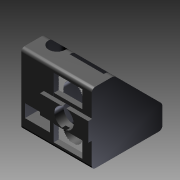
# Autodesk Inventor part: May Tec 1.64.153030.2_Mounting blocks GD-Zn_schwarz 0
Saved by Autodesk Inventor 2016 (Build 200138000, 138)
## iProperties
Category: PARTsolutions
Company: MAYTEC
Created: 2012-11-14
Part Number: May Tec 1.64.153030.2_Mounting blocks GD-Zn_schwarz 0
Catalog Web Link: www.cadenas.de
Description: 1.64.153030-Mounting block
Vendor: MAYTEC
Document SubType Name: Modeling
Designer: PARTuser1
Manufacturer: MAYTEC
Density: 1 g/cm^3
Material: Generic
Appearance: RGB(0.00000000000000,0.00000000000000,0.00000000000000)
Mass: 10.5528 g
Surface Area: 72.8477 cm^2
Volume: 10.5528 cm^3
PSOL_IDENT_0: {\\10.0.0.242\data_v9\23d-libs\maytec\maytec_3d\anbauzubehoer\befestigungsbloecke\befestigungsblock_
PSOL_IDENT_1: gd-zn.prj},254 {VTYP=3D},{NB=May Tec 1.64.153030.2_Mounting blocks GD-Zn_schwarz 0},{LINA=May Tec 1.
PSOL_IDENT_2: 64.153030.2_Mounting blocks GD-Zn_schwarz 0},{NN=1.64.153030},{DATE=14.09.2010 08:30:06},{GEOMDATE=0
PSOL_IDENT_3: 6.07.2009 00:00:00},{VERSION=},{LINEID=20},{LINESUBID=-1},{WBVAR=P}  {NB=May Tec 1.64.153030.2_Mount
PSOL_IDENT_4: ing blocks GD-Zn_schwarz 0},{LINA=May Tec 1.64.153030.2_Mounting blocks GD-Zn_schwarz 0},{KT=DUMMY},
PSOL_IDENT_5: {PARTNR=1.64.153030.2},{DESCRIPTION=Befestigungsblock GD-Zn},{B=30.0},{H=30.0},{L=30.0},{COLOR=schwa
PSOL_IDENT_6: rz},{COL=0.00,0.00,0.00,0.00},{XTRANS=Mounting blocks GD-Zn},{P=0}
CNS_NT: Mounting block
CNS_NB: May Tec 1.64.153030.2_Mounting blocks GD-Zn_schwarz 0
CNS_NBSYN: May Tec $PARTNR._$XTRANS._$COLOR. $P.
CNS_LINA: May Tec 1.64.153030.2_Mounting blocks GD-Zn_schwarz 0
CNS_PARTNR: 1.64.153030.2
CNS_DESCRIPTION: Mounting blocks GD-Zn
CNS_B: 30.0
CNS_H: 30.0
CNS_L: 30.0
CNS_COLOR: Black
CNS_COL: 0.00,0.00,0.00,0.00
CNS_XTRANS: Mounting blocks GD-Zn
CNS_P: 0
SUPPLIER: MAYTEC
ARTICLENO: May Tec 1.64.153030.2_Mounting blocks GD-Zn_schwarz 0
BOMINFO: May Tec 1.64.153030.2_Mounting blocks GD-Zn_schwarz 0
CREATOR: CADENAS GmbH
Title: May Tec 1.64.153030.2_Mounting blocks GD-Zn_schwarz 0
Author: Cadenas PARTsolutions
Comments: Mounting block
Autodesk Inventor part; units mm, degrees
sketch "Skizze_1" plane through (0, 0, 0) normal (1, 0, 0) x (0, 1, 0)
  arc A0 (1.5, 30) -> (0, 28.5) centre (1.5, 28.5) ccw
  line L0 (0, 28.5) -> (0, 1.5)
  arc A1 (0, 1.5) -> (1.5, 0) centre (1.5, 1.5) ccw
  line L1 (1.5, 0) -> (28.5, 0)
  arc A2 (28.5, 0) -> (30, 1.5) centre (28.5, 1.5) ccw
  line L2 (30, 1.5) -> (30, 8.4645)
  arc A3 (30, 8.4645) -> (29.2678, 10.2322) centre (27.5, 8.4645) ccw
  line L3 (29.2678, 10.2322) -> (10.2322, 29.2678)
  arc A4 (10.2322, 29.2678) -> (8.4645, 30) centre (8.4645, 27.5) ccw
  line L4 (8.4645, 30) -> (1.5, 30)
  constraints: 10 end point, 10 point on circle, 5 centre point
extrude "Extrusion1" add sketch "Skizze_1" along normal mid plane 30
sketch "Sketch2" plane through (15, 1.5, 0) normal (0, 0, -1) x (-1, 0, 0)
  point P0 (23.5, 21)
hole "Drilling 1" at (-8.5, 22.5, 0) direction (0, 0, 1) diameter 6.647 depth 12 countersink diameter 8 countersink angle 90 thread size "M8x1.25" class "6H" standard "ISO Metric profile"
sketch "Sketch3" plane through (-8.5, 22.5, 12) normal (0, 0, -1) x (-1, 0, 0)
  point P0 (0, 0)
hole "Drilling 2" at (-8.5, 22.5, 12) direction (0, 0, 1) diameter 10 depth 13
sketch "Skizze_5" plane through (0, 0, 30) normal (0, 0, 1) x (1, 0, 0)
  arc A0 (-12, 8.7) -> (-5, 8.7) centre (-8.5, 8.7) ccw
  line L0 (-5, 8.7) -> (-5, 12.9)
  arc A1 (-5, 12.9) -> (-12, 12.9) centre (-8.5, 12.9) ccw
  line L1 (-12, 12.9) -> (-12, 8.7)
  constraints: 4 end point, 4 point on circle, 2 centre point
extrude "Extrusion2" cut sketch "Skizze_5" against normal blind 30
sketch "Skizze_4" plane through (0, 0, 30) normal (0, 0, 1) x (1, 0, 0)
  line L0 (-2.4, 8) -> (12.1, 8)
  line L1 (12.1, 8) -> (12.1, 38)
  line L2 (12.1, 38) -> (-2.4, 38)
  line L3 (-2.4, 38) -> (-2.4, 8)
  constraints: 8 end point
extrude "Extrusion3" cut sketch "Skizze_4" against normal blind 24.1
sketch "Skizze_6" plane through (0, 0, 30) normal (0, 0, 1) x (1, 0, 0)
  arc A0 (0.75, 15.6) -> (8.95, 15.6) centre (4.85, 15.6) ccw
  line L0 (8.95, 15.6) -> (8.95, 20.6)
  arc A1 (8.95, 20.6) -> (0.75, 20.6) centre (4.85, 20.6) ccw
  line L1 (0.75, 20.6) -> (0.75, 15.6)
  constraints: 4 end point, 4 point on circle, 2 centre point
extrude "Extrusion4" cut sketch "Skizze_6" against normal blind 30
sketch "Skizze_8" plane through (0, 8, 0) normal (0, 1, 0) x (1, 0, 0)
  line L0 (4.9, -8) -> (4.9, -1)
  arc A0 (12, -8) -> (4.9, -1) centre (4.8281, -8.1737) ccw
  line L1 (12, -8) -> (4.9, -8)
  line L2 (4.9, -8) -> (4.9, -1)
  constraints: 6 end point, 2 point on circle, 1 centre point
revolve "Revolution1" cut sketch "Skizze_8" angle 180 about axis through (4.9, 8, 8) along (0, 0, 1)
sketch "Skizze_9" plane through (0, 0, 0) normal (0, 1, 0) x (-1, 0, 0)
  arc A0 (-0.8, 22.15) -> (-9, 22.15) centre (-4.9, 22.15) ccw
  line L0 (-9, 22.15) -> (-9, 7.85)
  arc A1 (-9, 7.85) -> (-0.8, 7.85) centre (-4.9, 7.85) ccw
  line L1 (-0.8, 7.85) -> (-0.8, 22.15)
  constraints: 4 end point, 4 point on circle, 2 centre point
extrude "Extrusion5" cut sketch "Skizze_9" along normal blind 30
sketch "Skizze_10" plane through (0, 0, 0) normal (0, 1, 0) x (-1, 0, 0)
  line L0 (1.2, 27.8) -> (-11, 27.8)
  line L1 (-11, 27.8) -> (-11, 2.2)
  line L2 (-11, 2.2) -> (1.2, 2.2)
  line L3 (1.2, 2.2) -> (1.2, 27.8)
  constraints: 8 end point
extrude "Extrusion6" cut sketch "Skizze_10" along normal blind 2
sketch "Skizze_11" plane through (0, 0, 0) normal (0, 1, 0) x (-1, 0, 0)
  line L0 (13.4, 5) -> (13.4, 10.5)
  line L1 (13.4, 10.5) -> (2.75, 10.5)
  line L2 (2.75, 10.5) -> (2.75, 5)
  line L3 (2.75, 5) -> (13.4, 5)
  constraints: 8 end point
extrude "Extrusion7" cut sketch "Skizze_11" along normal blind 17.65
sketch "Skizze_7" plane through (4.9, 0, 0) normal (1, 0, 0) x (0, 0, -1)
  line L0 (-27.8, 1.7273) -> (-2.2, 1.7273)
  line L1 (-2.2, 1.7273) -> (-2.2, 2.3)
  line L2 (-2.2, 2.3) -> (-2.5, 2)
  line L3 (-2.5, 2) -> (-2.75, 2.3)
  line L4 (-2.75, 2.3) -> (-3, 2)
  line L5 (-3, 2) -> (-3.25, 2.3)
  line L6 (-3.25, 2.3) -> (-3.5, 2)
  line L7 (-3.5, 2) -> (-3.75, 2.3)
  line L8 (-3.75, 2.3) -> (-4, 2)
  line L9 (-4, 2) -> (-4.25, 2.3)
  line L10 (-4.25, 2.3) -> (-4.5, 2)
  line L11 (-4.5, 2) -> (-4.75, 2.3)
  line L12 (-4.75, 2.3) -> (-5, 2)
  line L13 (-5, 2) -> (-5.25, 2.3)
  line L14 (-5.25, 2.3) -> (-5.5, 2)
  line L15 (-5.5, 2) -> (-5.75, 2.3)
  line L16 (-5.75, 2.3) -> (-6, 2)
  line L17 (-6, 2) -> (-6.25, 2.3)
  line L18 (-6.25, 2.3) -> (-6.5, 2)
  line L19 (-6.5, 2) -> (-6.75, 2.3)
  line L20 (-6.75, 2.3) -> (-7, 2)
  line L21 (-7, 2) -> (-7.25, 2.3)
  line L22 (-7.25, 2.3) -> (-7.5, 2)
  line L23 (-7.5, 2) -> (-7.75, 2.3)
  line L24 (-7.75, 2.3) -> (-8, 2)
  line L25 (-8, 2) -> (-8.25, 2.3)
  line L26 (-8.25, 2.3) -> (-8.5, 2)
  line L27 (-8.5, 2) -> (-8.75, 2.3)
  line L28 (-8.75, 2.3) -> (-9, 2)
  line L29 (-9, 2) -> (-9.25, 2.3)
  line L30 (-9.25, 2.3) -> (-9.5, 2)
  line L31 (-9.5, 2) -> (-9.75, 2.3)
  line L32 (-9.75, 2.3) -> (-10, 2)
  line L33 (-10, 2) -> (-10.25, 2.3)
  line L34 (-10.25, 2.3) -> (-10.5, 2)
  line L35 (-10.5, 2) -> (-10.75, 2.3)
  line L36 (-10.75, 2.3) -> (-11, 2)
  line L37 (-11, 2) -> (-11.25, 2.3)
  line L38 (-11.25, 2.3) -> (-11.5, 2)
  line L39 (-11.5, 2) -> (-11.75, 2.3)
  line L40 (-11.75, 2.3) -> (-12, 2)
  line L41 (-12, 2) -> (-12.25, 2.3)
  line L42 (-12.25, 2.3) -> (-12.5, 2)
  line L43 (-12.5, 2) -> (-12.75, 2.3)
  line L44 (-12.75, 2.3) -> (-13, 2)
  line L45 (-13, 2) -> (-13.25, 2.3)
  line L46 (-13.25, 2.3) -> (-13.5, 2)
  line L47 (-13.5, 2) -> (-13.75, 2.3)
  line L48 (-13.75, 2.3) -> (-14, 2)
  line L49 (-14, 2) -> (-14.25, 2.3)
  line L50 (-14.25, 2.3) -> (-14.5, 2)
  line L51 (-14.5, 2) -> (-14.75, 2.3)
  line L52 (-14.75, 2.3) -> (-15, 2)
  line L53 (-15, 2) -> (-15.25, 2.3)
  line L54 (-15.25, 2.3) -> (-15.5, 2)
  line L55 (-15.5, 2) -> (-15.75, 2.3)
  line L56 (-15.75, 2.3) -> (-16, 2)
  line L57 (-16, 2) -> (-16.25, 2.3)
  line L58 (-16.25, 2.3) -> (-16.5, 2)
  line L59 (-16.5, 2) -> (-16.75, 2.3)
  line L60 (-16.75, 2.3) -> (-17, 2)
  line L61 (-17, 2) -> (-17.25, 2.3)
  line L62 (-17.25, 2.3) -> (-17.5, 2)
  line L63 (-17.5, 2) -> (-17.75, 2.3)
  line L64 (-17.75, 2.3) -> (-18, 2)
  line L65 (-18, 2) -> (-18.25, 2.3)
  line L66 (-18.25, 2.3) -> (-18.5, 2)
  line L67 (-18.5, 2) -> (-18.75, 2.3)
  line L68 (-18.75, 2.3) -> (-19, 2)
  line L69 (-19, 2) -> (-19.25, 2.3)
  line L70 (-19.25, 2.3) -> (-19.5, 2)
  line L71 (-19.5, 2) -> (-19.75, 2.3)
  line L72 (-19.75, 2.3) -> (-20, 2)
  line L73 (-20, 2) -> (-20.25, 2.3)
  line L74 (-20.25, 2.3) -> (-20.5, 2)
  line L75 (-20.5, 2) -> (-20.75, 2.3)
  line L76 (-20.75, 2.3) -> (-21, 2)
  line L77 (-21, 2) -> (-21.25, 2.3)
  line L78 (-21.25, 2.3) -> (-21.5, 2)
  line L79 (-21.5, 2) -> (-21.75, 2.3)
  line L80 (-21.75, 2.3) -> (-22, 2)
  line L81 (-22, 2) -> (-22.25, 2.3)
  line L82 (-22.25, 2.3) -> (-22.5, 2)
  line L83 (-22.5, 2) -> (-22.75, 2.3)
  line L84 (-22.75, 2.3) -> (-23, 2)
  line L85 (-23, 2) -> (-23.25, 2.3)
  line L86 (-23.25, 2.3) -> (-23.5, 2)
  line L87 (-23.5, 2) -> (-23.75, 2.3)
  line L88 (-23.75, 2.3) -> (-24, 2)
  line L89 (-24, 2) -> (-24.25, 2.3)
  line L90 (-24.25, 2.3) -> (-24.5, 2)
  line L91 (-24.5, 2) -> (-24.75, 2.3)
  line L92 (-24.75, 2.3) -> (-25, 2)
  line L93 (-25, 2) -> (-25.25, 2.3)
  line L94 (-25.25, 2.3) -> (-25.5, 2)
  line L95 (-25.5, 2) -> (-25.75, 2.3)
  line L96 (-25.75, 2.3) -> (-26, 2)
  line L97 (-26, 2) -> (-26.25, 2.3)
  line L98 (-26.25, 2.3) -> (-26.5, 2)
  line L99 (-26.5, 2) -> (-26.75, 2.3)
  line L100 (-26.75, 2.3) -> (-27, 2)
  line L101 (-27, 2) -> (-27.25, 2.3)
  line L102 (-27.25, 2.3) -> (-27.5, 2)
  line L103 (-27.5, 2) -> (-27.8, 2.3)
  line L104 (-27.8, 2.3) -> (-27.8, 1.7273)
  constraints: 210 end point
extrude "Extrusion8" cut sketch "Skizze_7" along normal mid plane 12.2
sketch "Sketch_1" plane through (0, 0, 15) normal (0, 0, 1) x (1, 0, 0)
  line L0 (-5.35, 0) -> (-5.35, -1.7)
  line L1 (-5.35, -1.7) -> (15.15, -1.7)
  line L2 (15.15, -1.7) -> (15.15, 0)
  line L3 (15.15, 0) -> (-5.35, 0)
  constraints: 8 end point
extrude "Extrusion9" add sketch "Sketch_1" along normal mid plane 8
sketch "Sketch_4" plane through (4.9, 0, 0) normal (1, 0, 0) x (0, 0, -1)
  line L0 (-20.457, 0) -> (-9, 0)
  line L1 (-9, 0) -> (-9, 2.2)
  line L2 (-9, 2.2) -> (-20.457, 2.2)
  line L3 (-20.457, 2.2) -> (-20.457, 0)
  constraints: 8 end point
extrude "Extrusion10" add sketch "Sketch_4" along normal mid plane 12
sketch "Sketch14" plane through (-5.35, -1.7, 19) normal (0, -1, 0) x (1, 0, 0)
  point P0 (10.25, -4)
hole "Drilling 3" at (4.9, -1.7, 15) direction (0, 1, 0) diameter 8.2 depth 4
ref_plane "side_1_XY" through (5.1, 0, 15) normal (0, -1, 0) x (0, 0, 1)
ref_plane "side_1_YZ" through (5.1, 0, 15) normal (0, 0, 1) x (-1, 0, 0)
ref_plane "side_1_ZX" through (5.1, 0, 15) normal (-1, 0, 0) x (0, -1, 0)
ref_plane "side_2a_XY" through (5.1, 18.1, 0) normal (0, 0, -1) x (1, 0, 0)
ref_plane "side_2a_YZ" through (5.1, 18.1, 0) normal (1, 0, 0) x (0, -1, 0)
ref_plane "side_2a_ZX" through (5.1, 18.1, 0) normal (0, -1, 0) x (0, 0, -1)
ref_plane "side_2b_XY" through (-8.5, 22.5, 0) normal (0, 0, -1) x (1, 0, 0)
ref_plane "side_2b_YZ" through (-8.5, 22.5, 0) normal (1, 0, 0) x (0, -1, 0)
ref_plane "side_2b_ZX" through (-8.5, 22.5, 0) normal (0, -1, 0) x (0, 0, -1)
ref_plane "side_2c_XY" through (-8.5, 10.8, 0) normal (0, 0, -1) x (1, 0, 0)
ref_plane "side_2c_YZ" through (-8.5, 10.8, 0) normal (1, 0, 0) x (0, -1, 0)
ref_plane "side_2c_ZX" through (-8.5, 10.8, 0) normal (0, -1, 0) x (0, 0, -1)
body "Solid1"
